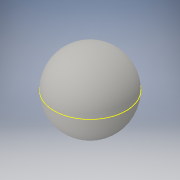
# Autodesk Inventor part: Aidan Sherry Marble
Saved by Autodesk Inventor 2016 (Build 200138000, 138)
## iProperties
Created: 2016-10-14
Part Number: Aidan Sherry Marble
Material: Generic
Document SubType Name: Modeling
Designer: sherra
Density: 1 g/cm^3
Appearance: Default
Author: sherra
Autodesk Inventor part; units mm, degrees
ref_plane "YZ Plane" through (0, 0, 0) normal (1, 0, 0) x (0, 1, 0)
ref_plane "XZ Plane" through (0, 0, 0) normal (0, 1, 0) x (-1, 0, 0)
ref_plane "XY Plane" through (0, 0, 0) normal (0, 0, 1) x (1, 0, 0)
sketch "Sketch3" plane through (0, 0, 0) normal (0, 0, 1) x (1, 0, 0)
  circle A0 centre (0, 0) radius 8.6995
  line L0 (0, 8.6995) -> (0, -8.6995)
  dimension "d3" = 17.399
  constraints: 2 end point, 2 point on circle, 1 centre point, 1 coincident, 1 vertical
  measures "d3" diameter of A0
revolve "Revolution1" add sketch "Sketch3" angle 360 about axis through (0, 8.6995, 0) along (0, -1, 0)
sketch "Sketch4" plane through (0, 0, 0) normal (0, 1, 0) x (-1, 0, 0)
  line L0 (0, -8.6818) -> (0, 8.6995)
  circle A0 centre (0, 0) radius 8.6995 projected
  constraints: 2 end point, 1 vertical, 1 vertical alignment, 1 other
body "Solid2"
